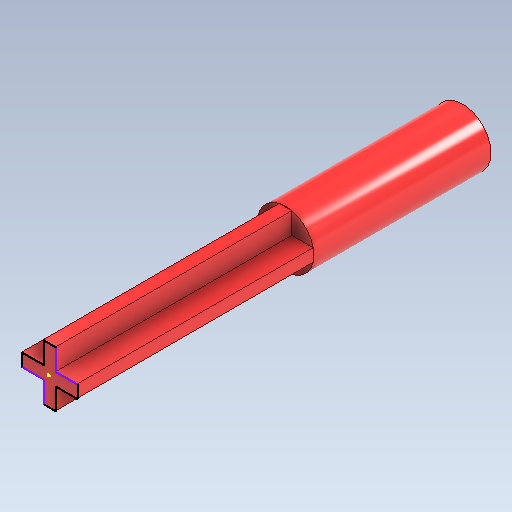
# Autodesk Inventor part: Bistable Rod
Saved by Autodesk Inventor 2020 (Build 240168000, 168)
## iProperties
Created: 2019-11-08
Part Number: Bistable Rod
Material: Generic
Document SubType Name: Modeling
Designer: camde
Density: 1 g/cm^3
Appearance: Light Red
Author: camde
Autodesk Inventor part; units mm, degrees
ref_plane "YZ Plane" through (0, 0, 0) normal (1, 0, 0) x (0, 1, 0)
ref_plane "XZ Plane" through (0, 0, 0) normal (0, 1, 0) x (-1, 0, 0)
ref_plane "XY Plane" through (0, 0, 0) normal (0, 0, 1) x (1, 0, 0)
sketch "Sketch1" plane through (0, 0, 0) normal (0, 0, 1) x (1, 0, 0)
  circle A0 centre (0, 0) radius 3.048
  dimension "d0" = 6.096
  constraints: 1 centre point, 1 coincident
  measures "d0" diameter of A0
extrude "Extrusion1" add sketch "Sketch1" along normal blind 38.1
sketch "Sketch2" plane through (0, 0, 0) normal (0, 0, -1) x (-1, 0, 0)
  circle A0 centre (0, 0) radius 3.048
  constraints: 1 centre point, 1 coincident
extrude "Extrusion2" cut sketch "Sketch2" against normal blind 6.35
sketch "Sketch3" plane through (0, 0, 6.35) normal (0, 0, -1) x (-1, 0, 0)
  circle A0 centre (0, 0) radius 3.048 projected
  line L0 (0, 0) -> (0, 0.6747) construction
  line L1 (-2.9727, 0.6731) -> (-0.6731, 0.6731)
  line L2 (0.6731, 0.6731) -> (2.9727, 0.6731)
  line L3 (-0.6731, 2.9727) -> (-0.6731, 0.6731)
  line L4 (-0.6731, -0.6731) -> (-0.6731, -2.9727)
  line L5 (0.6731, -2.9727) -> (0.6731, -0.6731)
  line L6 (0.6731, 0.6731) -> (0.6731, 2.9727)
  line L7 (-2.9727, -0.6731) -> (-0.6731, -0.6731)
  line L8 (0.6731, -0.6731) -> (2.9727, -0.6731)
  arc A1 (-0.6731, 2.9727) -> (-2.9727, 0.6731) centre (0, 0) ccw
  arc A2 (2.9727, 0.6731) -> (0.6731, 2.9727) centre (0, 0) ccw
  arc A3 (-2.9727, -0.6731) -> (-0.6731, -2.9727) centre (0, 0) ccw
  arc A4 (0.6731, -2.9727) -> (2.9727, -0.6731) centre (0, 0) ccw
  dimension "d5" = 1.3462
  constraints: 18 end point, 10 point on circle, 4 centre point, 4 horizontal, 4 parallel, 3 vertical, 1 coincident, 1 symmetric about line
  measures "d5" distance of L3.start L6.end
extrude "Extrusion3" cut sketch "Sketch3" against normal blind 31.75 contours L2 L6 A0 | A0 L5 L8 | L3 L1 A0 | A0 L7 L4
sketch "Sketch4" plane through (0, 0, 6.35) normal (0, 0, -1) x (-1, 0, 0)
  circle A0 centre (0, 0) radius 3.048 projected
  line L0 (-0.6731, 2.9727) -> (0.6731, 2.9727)
  line L1 (-2.9727, -0.6731) -> (-2.9727, 0.6731)
  line L2 (0.6731, -2.9727) -> (-0.6731, -2.9727)
  line L3 (2.9727, 0.6731) -> (2.9727, -0.6731)
  arc A1 (0.6731, 2.9727) -> (-0.6731, 2.9727) centre (0, 0) ccw
  arc A2 (2.9727, -0.6731) -> (2.9727, 0.6731) centre (0, 0) ccw
  arc A3 (-2.9727, 0.6731) -> (-2.9727, -0.6731) centre (0, 0) ccw
  arc A4 (-0.6731, -2.9727) -> (0.6731, -2.9727) centre (0, 0) ccw
  point P0 (-0.6731, -2.9727)
  point P1 (2.9727, -0.6731)
  point P2 (-2.9727, 0.6731)
  dimension "d14" = 360
  constraints: 10 point on circle, 8 end point, 4 centre point, 1 coincident, 1 horizontal, 13 other
extrude "Extrusion4" cut sketch "Sketch4" against normal blind 25.4 contours A0 L3 | L0 A0 | A0 L2 | L1 A0
sketch "Sketch5" plane through (0, 0, 6.35) normal (0, 0, -1) x (-1, 0, 0)
  circle A0 centre (0, 0) radius 3.048
  dimension "d18" = 6.096
  constraints: 1 centre point, 1 coincident
  measures "d18" diameter of A0
extrude "Extrusion5" add sketch "Sketch5" along normal blind 6.35
sketch "Sketch6" plane through (0, 0, 38.1) normal (0, 0, 1) x (1, 0, 0)
  circle A0 centre (0, 0) radius 3.048
  dimension "d21" = 6.096
  constraints: 1 centre point, 1 coincident
  measures "d21" diameter of A0
extrude "Extrusion6" cut sketch "Sketch6" against normal blind 6.35
sketch "Sketch7" plane through (0, 0, 31.75) normal (0, 0, 1) x (1, 0, 0)
  line L0 (-0.6731, 2.9727) -> (0.6731, 2.9727) projected
  line L1 (0.6731, -0.6731) -> (0.6731, -2.9727) projected
  line L2 (-0.6731, 2.9727) -> (0.6731, 2.9727)
  line L3 (0.6731, -2.9727) -> (-0.6731, -2.9727)
  line L4 (-2.9727, -0.6731) -> (-2.9727, 0.6731) projected
  line L5 (2.9727, -0.6731) -> (2.9727, -0.6731) projected
  line L6 (2.9727, 0.6731) -> (2.9727, -0.6731)
  line L7 (-2.9727, -0.6731) -> (-2.9727, 0.6731)
  line L8 (-2.9727, 0.6731) -> (-0.6731, 0.6731)
  line L9 (0.6731, 0.6731) -> (2.9727, 0.6731)
  line L10 (-0.6731, -2.9727) -> (-0.6731, -0.6731)
  line L11 (-0.6731, 0.6731) -> (-0.6731, 2.9727)
  line L12 (0.6731, 2.9727) -> (0.6731, 0.6731)
  line L13 (0.6731, -0.6731) -> (0.6731, -2.9727)
  line L14 (2.9727, -0.6731) -> (0.6731, -0.6731)
  line L15 (-0.6731, -0.6731) -> (-2.9727, -0.6731)
  point P0 (0, 0)
  constraints: 25 end point, 10 parallel, 4 perpendicular, 3 horizontal, 1 point on line
sketch "Sketch8" plane through (0, 0, 0) normal (0, 0, -1) x (-1, 0, 0)
  circle A0 centre (0, 0) radius 3.048
  constraints: 1 centre point, 1 coincident
extrude "Extrusion7" add sketch "Sketch8" along normal blind 12.7
body "Solid1"
